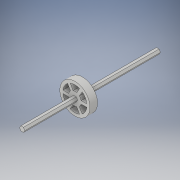
# Autodesk Inventor part: RobotArm HexWheel
Saved by Autodesk Inventor 2018 (Build 220112000, 112)
## iProperties
Created: 2018-01-13
Part Number: RobotArm HexWheel
Material: Generic
Document SubType Name: Modeling
Designer: lopez.xavier
Density: 1 g/cm^3
Appearance: Default
Author: lopez.xavier
Autodesk Inventor part; units mm, degrees
note: some values were not read from the file. Chosen so that the rebuilt part matches the saved one: sketch regions of "Extrusion3".
ref_plane "YZ Plane" through (0, 0, 0) normal (1, 0, 0) x (0, 1, 0)
ref_plane "XZ Plane" through (0, 0, 0) normal (0, 1, 0) x (-1, 0, 0)
sketch "Sketch1" plane through (0, 0, 0) normal (0, 0, 1) x (1, 0, 0)
  line L0 (2.1997, 3.81) -> (4.3994, 0)
  line L1 (4.3994, 0) -> (2.1997, -3.81)
  line L2 (2.1997, -3.81) -> (-2.1997, -3.81)
  line L3 (-2.1997, -3.81) -> (-4.3994, 0)
  line L4 (-4.3994, 0) -> (-2.1997, 3.81)
  line L5 (-2.1997, 3.81) -> (2.1997, 3.81)
  line L6 (0, 0) -> (1.0543, 0)
  dimension "d0" = 7.62
  constraints: 14 end point, 1 coincident, 1 horizontal, 1 parallel, 13 other
  measures "d0" distance between parallel lines of L2 L5
extrude "Extrusion1" add sketch "Sketch1" along normal blind 228.6
ref_plane "Work Plane1" through (0, 0, 127) normal (0, 0, 1) x (1, 0, 0)
sketch "Sketch2" plane through (0, 0, 127) normal (0, 0, 1) x (1, 0, 0)
  line L0 (2.1997, 3.81) -> (4.3994, 0) construction
  line L1 (4.3994, 0) -> (2.1997, -3.81) projected
  line L2 (2.1997, -3.81) -> (-2.1997, -3.81) projected
  line L3 (-2.1997, -3.81) -> (-4.3994, 0) projected
  line L4 (-4.3994, 0) -> (-2.1997, 3.81) projected
  line L5 (-2.1997, 3.81) -> (2.1997, 3.81) projected
  circle A0 centre (0, 0) radius 25.4
  circle A1 centre (0, 0) radius 20.32
  circle A2 centre (0, 0) radius 10.795
  line L6 (-2.1997, 3.81) -> (-4.3994, 0) projected
  line L7 (-4.3994, 0) -> (-2.1997, -3.81) projected
  line L8 (2.1997, -3.81) -> (4.3994, 0) projected
  line L9 (2.1997, 3.81) -> (-2.1997, 3.81) projected
  line L10 (4.3994, 0) -> (2.1997, 3.81) projected
  line L11 (-4.3994, 0) -> (-20.32, 0)
  line L12 (4.3994, 0) -> (20.32, 0)
  line L13 (10.4919, -2.54) -> (20.1606, -2.54)
  line L14 (10.4919, 2.54) -> (20.1606, 2.54)
  line L15 (-10.4919, 2.54) -> (-20.1606, 2.54)
  line L16 (-10.4919, -2.54) -> (-20.1606, -2.54)
  line L17 (-2.1997, 3.81) -> (-10.16, 17.5976)
  line L18 (2.1997, 3.81) -> (10.16, 17.5976)
  line L19 (-2.1997, -3.81) -> (2.1997, -3.81) projected
  line L20 (2.1997, -3.81) -> (10.16, -17.5976)
  line L21 (-2.1997, -3.81) -> (-10.16, -17.5976)
  line L22 (-7.4457, 7.8163) -> (-12.28, 16.1896)
  line L23 (-3.0463, 10.3563) -> (-7.8806, 18.7296)
  line L24 (3.0463, 10.3563) -> (7.8806, 18.7296)
  line L25 (7.4457, 7.8163) -> (12.28, 16.1896)
  line L26 (7.4457, -7.8163) -> (12.28, -16.1896)
  line L27 (3.0463, -10.3563) -> (7.8806, -18.7296)
  line L28 (-7.4457, -7.8163) -> (-12.28, -16.1896)
  line L29 (-3.0463, -10.3563) -> (-7.8806, -18.7296)
  dimension "d6" = 21.59
  dimension "d4" = 50.8
  dimension "d5" = 5.08
  dimension "d31" = 5.08
  dimension "d32" = 2.54
  dimension "d33" = 5.08
  dimension "d34" = 2.54
  dimension "d35" = 120
  dimension "d36" = 120
  dimension "d37" = 120
  dimension "d38" = 120
  dimension "d39" = 5.08
  dimension "d40" = 2.54
  dimension "d41" = 5.08
  dimension "d42" = 2.54
  dimension "d44" = 5.08
  dimension "d45" = 2.54
  dimension "d46" = 5.08
  dimension "d47" = 2.54
  constraints: 36 end point, 12 parallel, 3 coincident, 2 horizontal, 1 centre point, 34 other
  measures "d4" diameter of A0
  measures "d31" distance between parallel lines of L14 L13
  measures "d32" distance between parallel lines of L12 L14
  measures "d33" distance between parallel lines of L16 L15
  measures "d34" distance between parallel lines of L11 L16
  measures "d35" angle of L3 L21
  measures "d36" angle of L1 L20
  measures "d37" angle of L0 L18
  measures "d38" angle of L4 L17
  measures "d39" distance between parallel lines of L22 L23
  measures "d40" distance between parallel lines of L17 L23
  measures "d41" distance between parallel lines of L25 L24
  measures "d42" distance between parallel lines of L18 L24
  measures "d44" distance between parallel lines of L26 L27
  measures "d45" distance between parallel lines of L20 L26
  measures "d46" distance between parallel lines of L28 L29
  measures "d47" distance between parallel lines of L21 L29
extrude "Extrusion3" add sketch "Sketch2" along normal blind 12.7 contours L12 A2 L20 L1 | L10 L18 A2 L12 | L20 A2 L21 L2 | L5 L17 A2 L18 | L12 A1 L13 A2 | A2 L14 A1 L12 | L21 A2 L11 L3 | L20 A1 L27 A2 | A2 L26 A1 L20 | L4 L11 A2 L17 | L18 A1 L25 A2 | A2 L24 A1 L18 | L21 A1 L28 A2 | A2 L29 A1 L21 | L17 A1 L23 A2 | A2 L22 A1 L17 | L11 A1 L15 A2 | A2 L16 A1 L11 | A0
equation "\"d36\" = d35"
equation "\"d37\" = d35"
equation "\"d38\" = d35"
body "Solid1"
